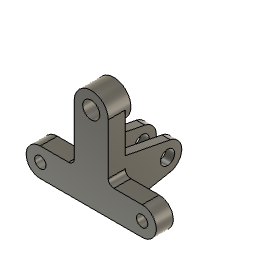
A2_AI22BTECH11005_3 (Autodesk Fusion 360 design; units mm, degrees)
Autodesk Fusion 360 part; units mm, degrees
sketch "Sketch2" plane through (0, 0, 0) normal (0, 1, 0) x (1, 0, 0)
  line L0 (-30, 0) -> (-30, 90)
  line L1 (30, 100) -> (30, 150)
  line L2 (30, 150) -> (90, 150)
  line L3 (30, 150) -> (-90, 150)
  line L4 (-90, 100) -> (-40, 100)
  arc A0 (-30, 90) -> (-40, 100) centre (-40, 90) ccw
  line L5 (40, 100) -> (90, 100)
  arc A1 (-30, 0) -> (30, 0) centre (0, 0) ccw
  arc A2 (30, 0) -> (-30, 0) centre (0, 0) ccw
  arc A3 (-15, 0) -> (15, 0) centre (0, 0) ccw
  arc A4 (15, 0) -> (-15, 0) centre (0, 0) ccw
  line L6 (30, 0) -> (30, 90)
  arc A5 (90, 100) -> (90, 150) centre (90, 125) ccw
  arc A6 (-90, 150) -> (-90, 100) centre (-90, 125) ccw
  arc A7 (40, 100) -> (30, 90) centre (40, 90) ccw
  circle A8 centre (-90, 125) radius 10
  circle A9 centre (90, 125) radius 10
  point P0 (-30, 150)
  dimension "d1" = 150
  dimension "d2" = 60
  dimension "d3" = 60
  dimension "d4" = 120
  dimension "d5" = 30
  dimension "d6" = 25
  dimension "d7" = 25
  dimension "d8" = 25
  dimension "d9" = 10
  dimension "d10" = 10
  dimension "d11" = 20
  dimension "d12" = 20
  constraint vertical L0
  constraint perpendicular L1 L2
  constraint perpendicular L0 L3
  constraint coincident A1.centre A2.centre
  constraint tangent L1 A1
  constraint concentric A1 A3
  constraint perpendicular L1 L4
  constraint coincident P0 L0
  constraint coincident L5.end L4
  constraint tangent L0 A0
  constraint tangent L4 A0
  constraint tangent L5 A5
  constraint concentric A1 A2
  constraint concentric A3 A4
  constraint coincident L1.start L5
  constraint tangent L6 A7
  constraint tangent L5 A7
  constraint concentric A6 A8
  constraint concentric A5 A9
  measures "d1" distance of L0.start P0
  measures "d2" distance of L0.start A1.end
  measures "d3" distance of L1.end L2.end
  measures "d4" distance of L1.end L3.end
  measures "d5" diameter of A3
  measures "d6" distance of L3.end A6.centre
  measures "d7" distance of L4.start A6.centre
  measures "d8" distance of L5.end A5.centre
  measures "d9" radius of A0
  measures "d10" radius of A7
  measures "d11" diameter of A8
  measures "d12" diameter of A9
extrude "Extrude1" add sketch "Sketch2" along normal blind 40 contours A1 A2
extrude "Extrude2" add sketch "Sketch2" along normal blind 30 contours L0 L2 L3 L4 A0 L5 A2 L6 A5 A6 A7
sketch "Sketch3" plane through (0, 30, 0) normal (0, 1, 0) x (-1, 0, 0)
  circle A0 centre (-90, -125) radius 10
  circle A1 centre (90, -125) radius 10
  arc A2 (-90, -100) -> (-90, -150) centre (-90, -125) ccw
  line L0 (-90, -150) -> (90, -150)
  arc A3 (90, -150) -> (90, -100) centre (90, -125) ccw
  line L1 (90, -100) -> (40, -100)
  arc A4 (30, -90) -> (40, -100) centre (40, -90) ccw
  line L2 (30, -90) -> (30, 0)
  arc A5 (-30, 0) -> (30, 0) centre (0, 0) ccw
  line L3 (-30, 0) -> (-30, -90)
  arc A6 (-40, -100) -> (-30, -90) centre (-40, -90) ccw
  line L4 (-40, -100) -> (-90, -100)
sketch "Sketch4" plane through (30, 0, 0) normal (1, 0, 0) x (0, 1, 0)
  line L0 (0, 0) -> (0, -90)
  line L1 (0, -90) -> (30, -90)
  line L2 (30, -90) -> (30, 0)
  line L3 (30, 0) -> (0, 0)
  line L4 (30, -150) -> (30, -70)
  line L5 (105, -84.5349) -> (105, -85)
  arc A0 (109.7565, -134.5434) -> (109.7565, -85.4566) centre (105, -110) ccw
  arc A1 (105, -122.5) -> (105, -97.5) centre (105, -110) ccw
  arc A2 (105, -97.5) -> (105, -122.5) centre (105, -110) ccw
  line L6 (30, -70) -> (109.7565, -85.4566)
  line L7 (30, -150) -> (109.7565, -134.5434)
  dimension "d17" = 80
  dimension "d20" = 25
  dimension "d24" = 0
  dimension "d25" = 0
  constraint perpendicular L1 L4
  constraint coincident A0.centre L5
  constraint concentric A1 A2
  constraint tangent A0 L6
  constraint tangent A0 L7
  constraint coincident L6 L5.start
  measures "d17" distance of L4.start L4.end
  measures "d20" diameter of A1
extrude "Extrude3" add sketch "Sketch4" against normal blind 15 contours L2 L4 A0 L6 L7
sketch "Sketch7" plane through (-30, 0, 0) normal (-1, 0, 0) x (0, -1, 0)
  line L0 (0, -90) -> (0, 0)
  line L1 (0, 0) -> (-30, 0)
  line L2 (-30, 0) -> (-30, -90)
  line L3 (-30, -90) -> (0, -90)
  line L4 (-30, -70) -> (-30, -150)
  circle A0 centre (-105, -110) radius 12.5
  line L5 (-105, -84.5349) -> (-109.7565, -85.4566)
  line L6 (-105, -135.4651) -> (-109.7565, -134.5434)
  line L7 (-30, -150) -> (-105, -135.4651)
  line L8 (-30, -70) -> (-105, -84.5349)
  arc A1 (-109.7565, -85.4566) -> (-109.7565, -134.5434) centre (-105, -110) ccw
  dimension "d29" = 25
  constraint coincident L2 L4.start
  measures "d29" diameter of A0
extrude "Extrude4" add sketch "Sketch7" against normal blind 15 contours L2 L4 L5 L6 L7 L8 A1
